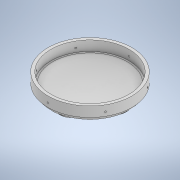
# Autodesk Inventor part: Main Mirror
Saved by Autodesk Inventor 2022 (Build 260153000, 153)
## iProperties
Created: 2023-08-20
Part Number: Main Mirror
Material: Generic
Document SubType Name: Modeling
Designer: fouad
Density: 1 g/cm^3
Appearance: Default
Author: fouad
Autodesk Inventor part; units mm, degrees
ref_plane "YZ Plane" through (0, 0, 0) normal (1, 0, 0) x (0, 1, 0)
ref_plane "XZ Plane" through (0, 0, 0) normal (0, 1, 0) x (-1, 0, 0)
ref_plane "XY Plane" through (0, 0, 0) normal (0, 0, 1) x (1, 0, 0)
sketch "Sketch2" plane through (0, 0, 0) normal (0, 0, 1) x (1, 0, 0)
  circle A0 centre (0, 0) radius 25
  circle A1 centre (0, 0) radius 24
  line L0 (-28.1544, -15) -> (30.7149, -15)
  line L1 (0, -25) -> (0, -24)
  point P0 (20, -15)
  point P1 (18.735, -15)
  dimension "d3" = 50
  dimension "d4" = 48
  dimension "d6" = 10
  constraints: 4 end point, 2 coincident, 1 horizontal, 1 perpendicular, 6 other
  measures "d6" distance from line of L0 L1.start
revolve "Revolution1" add sketch "Sketch2" angle 360 about axis through (0, -25, 0) along (0, 1, 0) picked at (16.5634, -17.6598) contours A0 L1 A1 L0
sketch "Sketch3" plane through (0, 0, 0) normal (0, 0, 1) x (1, 0, 0)
  arc A0 (-20, -15) -> (20, -15) centre (0, 0) ccw projected
  circle A1 centre (0, 0) radius 25
  circle A2 centre (0, 0) radius 25.875
  line L0 (20, -15) -> (21.0835, -15)
  line L1 (-20, -15) -> (20, -15) projected
  line L2 (0, -15) -> (0, -25)
  line L3 (-20, -15) -> (-21.0835, -15)
  line L4 (0, -25.875) -> (0, -25)
  line L5 (-38.5, 0) -> (38.5, 0) projected
  line L6 (0, -38.5) -> (0, 38.5) projected
  point P0 (20, -15)
  dimension "d7" = 51.75
  constraints: 8 end point, 5 point on circle, 2 centre point, 2 coincident, 2 symmetric about line, 1 horizontal, 1 midpoint, 1 vertical
  measures "d7" diameter of A2
revolve "Revolution2" add sketch "Sketch3" angle 360 about axis through (0, -10, 0) along (0, 1, 0) contours A0 L0 A2 L4
sketch "Sketch4" plane through (0, 0, 0) normal (0, 0, 1) x (1, 0, 0)
  line L0 (19.6202, -16.869) -> (18.4509, -16.869)
  line L1 (0, -25.875) -> (0, -25)
  line L2 (1.3306, -24.9646) -> (1.3306, -25.8408)
  line L3 (-19.6202, -16.869) -> (-18.4509, -16.869)
  line L4 (-1.3306, -24.9646) -> (-1.3306, -25.8408)
  circle A0 centre (0, 0) radius 25
  circle A1 centre (0, 0) radius 25.875
  line L5 (0, -36.225) -> (0, 36.225) projected
  constraints: 10 end point, 4 symmetric about line, 2 coincident, 1 horizontal, 1 vertical, 6 other
revolve "Revolution4" cut sketch "Sketch4" angle 80 about axis through (0, -10, 0) along (0, -1, 0) contours A1 L2 A0 L0
pattern_circular "Circular Pattern2" count 4 over 360 about axis through (0, -10, 0) along (0, 1, 0) of "Revolution4"
sketch "Sketch6" plane through (0, -15, 0) normal (0, 1, 0) x (1, 0, 0)
  line L0 (-19.6202, 0) -> (-1.3306, 0) projected
  circle A0 centre (0, 0) radius 19.6202
  circle A1 centre (0, 0) radius 21.0835 projected
  circle A2 centre (0, 0) radius 21.0835
  constraints: 2 coincident, 1 centre point, 1 horizontal alignment, 2 other
extrude "Extrusion3" add sketch "Sketch6" along normal blind 5
sketch "Sketch7" plane through (0, 0, 0) normal (0, 0, 1) x (1, 0, 0)
  line L0 (-21.0835, -15) -> (21.0835, -15) projected
  circle A0 centre (0, -13) radius 0.375
  point P0 (0, 0)
  dimension "d24" = 0.75
  dimension "d26" = 2
  constraints: 1 centre point
  measures "d24" diameter of A0
  measures "d26" distance from line of L0 A0.centre
extrude "Extrusion4" cut sketch "Sketch7" against normal through all
pattern_circular "Circular Pattern3" count 6 over 360 about axis through (0, -10, 0) along (0, 1, 0) of "Extrusion4"
body "Solid2"
